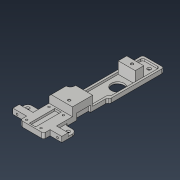
# Autodesk Inventor part: Kameraplatte
Saved by Autodesk Inventor 2022.1 (Build 261234020, 234B)
## iProperties
Part Number: Kameraplatte
Material: Aluminium 6061
Document SubType Name: Modeling
Designer: rYan
Mass: 35.1159 g
Surface Area: 82.272 cm^2
Volume: 13.0059 cm^3
Density: 2.7 g/cm^3
Appearance: Aluminium - flach
Author: rYan
Autodesk Inventor part; units mm, degrees
note: some values were not read from the file. Chosen so that the rebuilt part matches the saved one: direction of "Bohrung4".
ref_plane "YZ Plane" through (0, 0, 0) normal (1, 0, 0) x (0, 1, 0)
ref_plane "XZ Plane" through (0, 0, 0) normal (0, 1, 0) x (-1, 0, 0)
ref_plane "XY Plane" through (0, 0, 0) normal (0, 0, 1) x (1, 0, 0)
sketch "Skizze1" plane through (0, 0, 0) normal (0, 0, 1) x (1, 0, 0)
  line L0 (0, 102.2) -> (0, -102.2) projected
  line L1 (-33.3598, 0) -> (33.3598, 0) projected
  line L2 (14, 73) -> (-10, 73)
  line L3 (14, -73) -> (-10, -73)
  line L4 (-10, -53) -> (-19, -53)
  line L5 (-10, -61) -> (-23, -61)
  arc A0 (-19, -53) -> (-23, -57) centre (-19, -57) ccw
  line L6 (14, -53) -> (19, -53)
  line L7 (14, -61) -> (23, -61)
  arc A1 (23, -57) -> (19, -53) centre (19, -57) ccw
  line L8 (-10, -73) -> (-10, -61)
  line L9 (-10, -53) -> (-10, 73)
  line L10 (14, 73) -> (14, -53)
  line L11 (14, -61) -> (14, -73)
  line L12 (-23, -61) -> (-23, -57)
  line L13 (23, -61) -> (23, -57)
  point P0 (0, 0)
  dimension "d45" = 73
  dimension "d46" = 73
  dimension "d53" = 14
  dimension "d54" = 10
  dimension "d55" = 8
  dimension "d59" = 57
  dimension "d61" = 38
  constraints: 24 end point, 6 tangent, 4 collinear, 4 parallel, 4 point on circle, 3 horizontal, 2 centre point, 2 perpendicular, 2 vertical, 1 symmetric about line
  measures "d45" distance between parallel lines of L2 L1
  measures "d46" distance between parallel lines of L3 L1
  measures "d53" distance between parallel lines of L0 L11
  measures "d54" distance between parallel lines of L8 L0
  measures "d55" distance between parallel lines of L7 L6
  measures "d59" distance from line of L1 A0.centre
  measures "d61" distance of A1.centre A0.centre
extrude "Extrusion1" add sketch "Skizze1" along normal blind 2
sketch "Skizze4" plane through (0, 0, 2) normal (0, 0, 1) x (1, 0, 0)
  line L0 (-10, 73) -> (-10, -53) projected
  line L1 (0, 102.2) -> (0, -102.2) projected
  line L2 (-32.2, 0) -> (32.2, 0) projected
  line L3 (-10, 46) -> (-6, 46)
  line L4 (-6, 46) -> (-6, -30)
  line L5 (-6, -30) -> (-10, -30)
  line L6 (-10, -30) -> (-10, 46)
  line L7 (19, -53) -> (14, -53) projected
  line L8 (14, -53) -> (12, -53)
  line L9 (12, -53) -> (12, -13)
  line L10 (12, -13) -> (14, -13)
  line L11 (14, -13) -> (14, -53)
  line L12 (14, -73) -> (14, -61) projected
  line L13 (-10, -73) -> (14, -73) projected
  line L14 (14, -73) -> (12, -73)
  line L15 (12, -73) -> (12, -61)
  line L16 (12, -61) -> (14, -61)
  line L17 (14, -61) -> (14, -73)
  point P0 (0, 0)
  dimension "d62" = 4
  dimension "d81" = 46
  dimension "d82" = 30
  dimension "d158" = 2
  dimension "d159" = 40
  constraints: 24 end point, 6 parallel, 3 horizontal, 3 perpendicular, 2 point on line, 1 collinear
  measures "d62" distance of L3.start L3.end
  measures "d81" distance between parallel lines of L2 L3
  measures "d82" distance between parallel lines of L5 L2
  measures "d158" distance of L9.end L10.end
  measures "d159" distance of L8.end L9.end
extrude "Extrusion2" cut sketch "Skizze4" against normal through all
sketch "Skizze6" plane through (0, 0, 2) normal (0, 0, 1) x (1, 0, 0)
  line L0 (-6, -30) -> (-10, -30) projected
  line L1 (-10, -30) -> (-10, -53) projected
  line L2 (-10, -53) -> (-19, -53) projected
  arc A0 (-19, -53) -> (-23, -57) centre (-19, -57) ccw projected
  line L3 (-23, -61) -> (-10, -61) projected
  line L4 (-10, -61) -> (-10, -73) projected
  line L5 (-10, -73) -> (12, -73) projected
  line L6 (12, -61) -> (23, -61) projected
  arc A1 (23, -57) -> (19, -53) centre (19, -57) ccw projected
  line L7 (19, -53) -> (12, -53) projected
  line L8 (14, -13) -> (14, 73) projected
  line L9 (14, 73) -> (-10, 73) projected
  line L10 (-10, 73) -> (-10, 46) projected
  line L11 (-10, 46) -> (-6, 46) projected
  line L12 (-6, 46) -> (-6, -30) projected
  line L13 (-10, -73) -> (14, -73) projected
  line L14 (14, -53) -> (14, 73) projected
  line L15 (-10, -73) -> (12, -73)
  line L16 (12, -73) -> (12, -30)
  line L17 (12, -30) -> (-10, -30)
  line L18 (-10, -30) -> (-10, -73)
  line L19 (14, 73) -> (-10, 73) projected
  line L20 (-10, 73) -> (14, 73)
  line L21 (14, 73) -> (14, 46)
  line L22 (14, 46) -> (-10, 46)
  line L23 (-10, 46) -> (-10, 73)
  line L24 (-6, -30) -> (12, -30)
  line L25 (12, -30) -> (12, -27)
  line L26 (12, -27) -> (-6, -27)
  line L27 (-6, -27) -> (-6, -30)
  line L28 (-23, -57) -> (-23, -61) projected
  line L29 (23, -61) -> (23, -57) projected
  line L30 (12, -13) -> (14, -13) projected
  line L31 (12, -53) -> (12, -13) projected
  line L32 (12, -53) -> (12, -13) projected
  line L33 (12, -73) -> (12, -61) projected
  point P0 (0, 0)
  dimension "d83" = 27
  constraints: 24 end point, 6 parallel, 3 horizontal, 3 perpendicular, 3 point on line, 2 collinear
  measures "d83" distance from line of L26 point (0, 0)
extrude "Extrusion3" add sketch "Skizze6" along normal blind 3 contours L17 L16 L5 L4 L18 L1 L0 | L12 L26 L25 L17 | L11 L10 L9 L8 L22
sketch "Skizze7" plane through (0, 0, 5) normal (0, 0, 1) x (1, 0, 0)
  line L0 (12, -27) -> (-6, -27) projected
  line L1 (-6, -27) -> (-6, -30) projected
  line L2 (-6, -30) -> (-10, -30) projected
  line L3 (-10, -30) -> (-10, -73) projected
  line L4 (-10, -73) -> (12, -73) projected
  line L5 (-6, -27) -> (12, -27)
  line L6 (-6, -30) -> (-6, 46) projected
  line L7 (12, -27) -> (-6, -27) projected
  line L8 (12, -27) -> (12, -46)
  line L9 (14, -13) -> (14, 73) projected
  line L10 (12, -46) -> (-10, -46)
  line L11 (-10, -30) -> (-10, -53) projected
  line L12 (-10, -46) -> (-10, -30)
  line L13 (-10, -30) -> (-6, -30) projected
  line L14 (-10, -30) -> (-6, -30)
  line L15 (-6, -30) -> (-6, -27)
  line L16 (12, -73) -> (12, -27) projected
  point P0 (0, 0)
  dimension "d78" = 46
  constraints: 12 end point, 3 perpendicular, 2 collinear, 2 point on line, 1 other
  measures "d78" distance from line of point (0, 0) L10
extrude "Extrusion4" add sketch "Skizze7" along normal blind 8 contours L8 L10 L3 L2 L1 L0
sketch "Skizze8" plane through (0, 0, 2) normal (0, 0, 1) x (1, 0, 0)
  line L0 (14, 46) -> (-6, 46) projected
  line L1 (-6, 46) -> (-6, -27) projected
  line L2 (14, -13) -> (14, 46) projected
  line L3 (-6, -27) -> (12, -27) projected
  line L4 (14, 46) -> (12, 46)
  line L5 (12, 46) -> (12, -13)
  line L6 (12, -13) -> (14, -13)
  line L7 (14, -13) -> (14, 46)
  line L8 (-6, 46) -> (-6, -30) projected
  line L9 (-6, 46) -> (-4, 46)
  line L10 (-4, 46) -> (-4, -27)
  line L11 (-4, -27) -> (-6, -27)
  line L12 (-6, -27) -> (-6, 46)
  line L13 (-10, -53) -> (-19, -53) projected
  arc A0 (-19, -53) -> (-23, -57) centre (-19, -57) ccw projected
  line L14 (-23, -57) -> (-23, -61) projected
  line L15 (-23, -61) -> (-10, -61) projected
  line L16 (12, -61) -> (23, -61) projected
  line L17 (23, -61) -> (23, -57) projected
  arc A1 (23, -57) -> (19, -53) centre (19, -57) ccw projected
  line L18 (19, -53) -> (12, -53) projected
  line L19 (12, -13) -> (14, -13) projected
  line L20 (12, -27) -> (12, -13) projected
  line L21 (-6, -27) -> (12, -27) projected
  line L22 (-10, -61) -> (-10, -53) projected
  line L23 (12, -27) -> (10, -27)
  line L24 (10, -27) -> (10, -11)
  line L25 (10, -11) -> (12, -11)
  line L26 (12, -11) -> (12, -27)
  line L27 (12, -53) -> (12, -61) projected
  point P0 (0, 0)
  dimension "d84" = 2
  dimension "d160" = 2
  dimension "d161" = 2
  dimension "d162" = 2
  constraints: 25 end point, 6 parallel, 3 collinear, 3 horizontal, 3 perpendicular
  measures "d84" distance between parallel lines of L1 L10
  measures "d160" distance between parallel lines of L2 L5
  measures "d161" distance between parallel lines of L25 L6
  measures "d162" distance of L24.end L25.end
extrude "Extrusion5" add sketch "Skizze8" along normal blind 2 contours L2 L6 L5 L0 | L10 L3 L1 L0 | L5 L20 L3 L24 L25
sketch "Skizze2" plane through (0, 0, 2) normal (0, 0, 1) x (1, 0, 0)
  line L0 (-33.3598, 0) -> (33.3598, 0) projected
  line L1 (0, 102.2) -> (0, -102.2) projected
  arc A0 (-19, -53) -> (-23, -57) centre (-19, -57) ccw projected
  arc A1 (23, -57) -> (19, -53) centre (19, -57) ccw projected
  point P0 (0, 0)
  point P1 (6, 32)
  dimension "d50" = 32
  dimension "d60" = 6
  constraints: 2 coincident
  measures "d50" distance from line of point (6, 32) L0
  measures "d60" distance from line of point (6, 32) L1
hole "Bohrung1" at (19, -57, 2) at (6, 32, 2) at (-19, -57, 2) direction (0, 0, -1) diameter 3.3 end through all
sketch "Skizze3" plane through (0, 0, 2) normal (0, 0, 1) x (1, 0, 0)
  line L0 (-7, 70) -> (6.5, 70) construction
  line L1 (6.5, 70) -> (6.5, 49) construction
  line L2 (6.5, 49) -> (-7, 49) construction
  line L3 (-7, 49) -> (-7, 70) construction
  line L4 (-7, -49) -> (6.5, -49) construction
  line L5 (6.5, -49) -> (6.5, -70) construction
  line L6 (6.5, -70) -> (-7, -70) construction
  line L7 (-7, -70) -> (-7, -49) construction
  line L8 (0, 102.2) -> (0, -102.2) projected
  line L9 (-19, -60) -> (19, -60) projected
  line L10 (43, 45) -> (-43, 45) projected
  line L11 (-60.2, 0) -> (60.2, 0) projected
  point P0 (0, 0)
  dimension "d24" = 13.5
  dimension "d25" = 21
  dimension "d26" = 13.5
  dimension "d27" = 21
  dimension "d28" = 7
  dimension "d29" = 7
  dimension "d43" = 49
  constraints: 16 end point, 8 coincident, 4 parallel, 2 horizontal, 2 perpendicular, 1 other
  measures "d24" distance of L1.end L2.end
  measures "d25" distance of L0.end L1.end
  measures "d26" distance of L5.end L6.end
  measures "d27" distance of L4.end L5.end
  measures "d28" distance between parallel lines of L3 L8
  measures "d29" distance between parallel lines of L7 L8
  measures "d43" distance between parallel lines of L11 L4
hole "Bohrung2" at (-7, 70, 2) at (6.5, 70, 2) at (6.5, 49, 2) at (-7, 49, 2) at (-7, -49, 2) at (6.5, -49, 2) at (6.5, -70, 2) at (-7, -70, 2) direction (0, 0, -1) diameter 1.85 end through all both
fillet "Rundung3" radius 2 10 edges at (-10, -73, 2.5) (14, 73, 2.5) (-10, 73, 2.5) (-10, 46, 2.5) (-6, 46, 2) (-6, -30, 6.5) (-10, -30, 6.5) (-10, -53, 1) (12, -73, 2.5) (12, -53, 1)
sketch "Skizze9" plane through (14, -61, 0) normal (0, -1, 0) x (1, 0, 0)
  line L0 (-37, 0) -> (-24, 0) projected
  line L1 (-24, 0) -> (-24, 2) projected
  line L2 (-37, 2) -> (-24, 2) projected
  line L3 (-37, 0) -> (-37, 2) projected
  line L4 (9, 0) -> (9, 2) projected
  line L5 (-24, 5) -> (-22, 5) projected
  line L6 (-37, 0) -> (-24, 0)
  line L7 (-24, 0) -> (-24, 5)
  line L8 (-24, 5) -> (-37, 5)
  line L9 (-37, 5) -> (-37, 0)
  line L10 (9, 0) -> (-2, 0)
  line L11 (-2, 5) -> (9, 5)
  line L12 (9, 5) -> (9, 0)
  line L13 (-2, 0) -> (-2, 5)
  line L14 (9, 0) -> (-2, 0) projected
  line L15 (-2, 2) -> (9, 2) projected
  line L16 (-2, 2) -> (-2, 0) projected
  point P0 (-14, 0)
  dimension "d8" = 0
  constraints: 16 end point, 3 parallel, 2 collinear, 2 horizontal, 1 perpendicular
extrude "Extrusion6" add sketch "Skizze9" along normal blind 6
sketch "Skizze11" plane through (14, -67, 0) normal (0, -1, 0) x (1, 0, 0)
  line L0 (-33, 2) -> (5, 2) construction
  line L1 (-37, 0) -> (-37, 2) projected
  line L2 (-31.35, 0) -> (-34.65, 0) projected
  line L3 (-34.65, 2) -> (-31.35, 2) projected
  line L4 (6.65, 0) -> (3.35, 0) projected
  line L5 (3.35, 2) -> (6.65, 2) projected
  point P0 (-14, 0)
  dimension "d94" = 38
  constraints: 2 end point, 1 horizontal, 1 midpoint, 1 point on line
  measures "d94" distance of L0.start L0.end
hole "Bohrung4" at (19, -67, 2) at (-19, -67, 2) direction (0, 1, 0) diameter 1.85 depth 6
sketch "Skizze12" plane through (0, 0, 2) normal (0, 0, 1) x (1, 0, 0)
  line L0 (0, 102.2) -> (0, -102.2) projected
  line L1 (-32.2, 0) -> (32.2, 0) projected
  point P0 (0, 0)
  point P1 (6, 2.5)
  dimension "d102" = 6
  dimension "d103" = 2.5
  measures "d102" distance from line of point (6, 2.5) L0
  measures "d103" distance from line of point (6, 2.5) L1
hole "Bohrung5" at (6, 2.5, 2) direction (0, 0, -1) diameter 12 end through all
sketch "Skizze13" plane through (0, 0, 5) normal (0, 0, 1) x (1, 0, 0)
  circle A0 centre (-7, 70) radius 0.925 projected
  circle A1 centre (6.5, 70) radius 0.925 projected
  circle A2 centre (6.5, 49) radius 0.925 projected
  circle A3 centre (-7, 49) radius 0.925 projected
  circle A4 centre (6.5, -49) radius 0.925 projected
  circle A5 centre (-7, -49) radius 0.925 projected
  circle A6 centre (-7, -70) radius 0.925 projected
  circle A7 centre (6.5, -70) radius 0.925 projected
  circle A8 centre (6.5, -70) radius 0.925 construction
  line L0 (-7, -49) -> (6.5, -49) construction
  line L1 (6.5, -49) -> (6.5, -70) construction
  line L2 (6.5, -70) -> (-7, -70) construction
  line L3 (-7, -70) -> (-7, -49) construction
  circle A9 centre (-7, 70) radius 0.925 construction
  circle A10 centre (6.5, 49) radius 0.925 construction
  line L4 (-7, 70) -> (6.5, 70) construction
  line L5 (6.5, 70) -> (6.5, 49) construction
  line L6 (6.5, 49) -> (-7, 49) construction
  line L7 (-7, 49) -> (-7, 70) construction
  line L8 (-3, -47.5) -> (3, -47.5)
  line L9 (3, -47.5) -> (3, -71.5)
  line L10 (3, -71.5) -> (-3, -71.5)
  line L11 (-3, -71.5) -> (-3, -47.5)
  line L12 (-3, 71.5) -> (3, 71.5)
  line L13 (3, 71.5) -> (3, 47.5)
  line L14 (3, 47.5) -> (-3, 47.5)
  line L15 (-3, 47.5) -> (-3, 71.5)
  line L16 (0, 102.2) -> (0, -102.2) projected
  point P0 (0, 0)
  dimension "d115" = 1.5
  dimension "d116" = 1.5
  dimension "d117" = 6
  dimension "d118" = 1.5
  dimension "d119" = 1.5
  constraints: 32 end point, 8 parallel, 4 horizontal, 4 perpendicular, 1 point on line, 2 other
  measures "d115" distance between parallel lines of L8 L0
  measures "d116" distance between parallel lines of L10 L2
  measures "d117" distance of L8.start L8.end
  measures "d118" distance between parallel lines of L6 L14
  measures "d119" distance between parallel lines of L12 L4
extrude "Extrusion7" cut sketch "Skizze13" against normal blind 2 contours L8 L16 L10 L11 | L8 L9 L10 L16 | L12 L16 L14 L15 | L12 L13 L14 L16
sketch "Skizze14" plane through (0, 0, 5) normal (0, 0, 1) x (1, 0, 0)
  line L0 (-17.0333, 38) -> (20.6392, 38)
  line L1 (20.6392, 38) -> (20.6392, 88.9456)
  line L2 (20.6392, 88.9456) -> (-17.0333, 88.9456)
  line L3 (-17.0333, 88.9456) -> (-17.0333, 38)
  arc A0 (-6, 44) -> (-8, 46) centre (-8, 44) ccw projected
  point P0 (0, 0)
  dimension "d126" = 6
  constraints: 8 end point, 2 parallel, 1 horizontal, 1 perpendicular
  measures "d126" distance from line of L0 A0.centre
extrude "Extrusion8" cut sketch "Skizze14" against normal through all
sketch "Skizze15" plane through (0, 0, 2) normal (0, 0, 1) x (1, 0, 0)
  line L0 (12, 38) -> (-4, 38) projected
  line L1 (-4, 38) -> (-4, -27) projected
  line L2 (-4, -27) -> (10, -27) projected
  line L3 (12, -11) -> (12, 2.5) projected
  circle A0 centre (6, 2.5) radius 6 projected
  line L4 (12, 2.5) -> (12, 38) projected
  circle A1 centre (6, 32) radius 1.65 projected
  line L5 (12, 2.5) -> (12, 38) projected
  line L6 (-4, 38) -> (-4, -27) projected
  line L7 (12, 38) -> (-4, 38)
  line L8 (-4, 38) -> (-4, 36)
  line L9 (-4, 36) -> (12, 36)
  line L10 (12, 36) -> (12, 38)
  line L11 (12, -51) -> (12, -61) projected
  line L12 (23, -61) -> (23, -57) projected
  arc A2 (23, -57) -> (19, -53) centre (19, -57) ccw projected
  line L13 (19, -53) -> (14, -53) projected
  line L14 (10, -27) -> (10, -11) projected
  line L15 (10, -11) -> (12, -11) projected
  line L16 (12, -61) -> (18.075, -61) projected
  line L17 (18.075, -61) -> (19.925, -61) projected
  line L18 (19.925, -61) -> (23, -61) projected
  arc A3 (12, -51) -> (14, -53) centre (14, -51) ccw projected
  point P0 (0, 0)
  dimension "d123" = 2
  constraints: 8 end point, 2 parallel, 1 horizontal, 1 horizontal alignment, 1 perpendicular, 1 point on line
  measures "d123" distance between parallel lines of L0 L9
extrude "Extrusion9" add sketch "Skizze15" along normal blind 2 contours L4 L9 L1 L0
fillet "Rundung5" radius 2 8 edges at (14, 38, 2) (-6, 38, 2) (-4, 36, 3) (12, 36, 3) (14, -13, 2) (12, -13, 2) (12, -11, 3) (10, -11, 3)
sketch "Skizze18" plane through (12, -53, 2) normal (1, 0, 0) x (0, 0, -1)
  line L0 (2, 21) -> (2, 2) projected
  line L1 (2, 11) -> (-4, 11)
  line L2 (-4, 11) -> (-4, 24)
  line L3 (-4, 24) -> (2, 24)
  line L4 (2, 24) -> (2, 11)
  line L5 (0, 0) -> (2, 0) projected
  line L6 (2, 0) -> (0, 0) projected
  point P0 (2, 53)
  dimension "d164" = 13
  dimension "d165" = 6
  dimension "d192" = 11
  constraints: 8 end point, 2 parallel, 1 horizontal, 1 perpendicular, 1 point on line
  measures "d164" distance of L1.end L2.end
  measures "d165" distance of L2.end L3.end
  measures "d192" distance between parallel lines of L1 L5
extrude "Extrusion10" cut sketch "Skizze18" against normal blind 2
chamfer "Fase3" distance 2 angle 45 1 edges at (10, -35.5, 6)
chamfer "Fase4" distance 0.3 angle 45 4 edges at (19, -55.35, 0) (-19, -55.35, 0) (6, 8.5, 0) (6, 33.65, 0)
sketch "Skizze19" plane through (0, 0, 2) normal (0, 0, 1) x (1, 0, 0)
  arc A0 (11, -10.7321) -> (12, -9) centre (10, -9) ccw projected
  line L0 (12, -9) -> (12, 2.5) projected
  circle A1 centre (6, 2.5) radius 6 projected
  line L1 (12, 2.5) -> (12, 34) projected
  arc A2 (12, 34) -> (10, 36) centre (10, 34) ccw projected
  line L2 (10, 36) -> (-2, 36) projected
  arc A3 (-2, 36) -> (-4, 34) centre (-2, 34) ccw projected
  line L3 (-4, 34) -> (-4, -27) projected
  line L4 (-4, -27) -> (10, -27) projected
  line L5 (10, -27) -> (10, -12.4641) projected
  arc A4 (11, -10.7321) -> (10, -12.4641) centre (12, -12.4641) ccw projected
  circle A5 centre (6, 32) radius 1.65 projected
  line L6 (-4, 34) -> (-4, -27) projected
  line L7 (12, 13) -> (-4, 13)
  line L8 (-4, 13) -> (-4, 21)
  line L9 (-4, 21) -> (12, 21)
  line L10 (12, 21) -> (12, 13)
  point P0 (0, 0)
  dimension "d174" = 8
  dimension "d175" = 13
  constraints: 8 end point, 2 parallel, 2 point on line, 1 horizontal, 1 horizontal alignment, 1 perpendicular
  measures "d174" distance between parallel lines of L9 L7
  measures "d175" distance from line of point (0, 0) L7
extrude "Extrusion11" add sketch "Skizze19" along normal up to surface (11 mm away) contours L7 L3 L9 L1
sketch "Skizze5" plane through (0, 0, 2) normal (0, 0, 1) x (1, 0, 0)
  line L0 (0, 102.2) -> (0, -102.2) projected
  point P0 (0, 0)
  point P1 (0, -33)
  point P2 (0, -40)
  dimension "d66" = 7
  dimension "d67" = 33
  constraints: 2 point on line
  measures "d66" distance of point (0, -40) point (0, -33)
  measures "d67" distance of point (0, 0) point (0, -33)
hole "Bohrung3" [suppressed]
sketch "Skizze20" plane through (0, 0, 13) normal (0, 0, 1) x (1, 0, 0)
  point P0 (0, 0)
  point P1 (5, -42)
  point P2 (5, 17)
  dimension "d178" = 42
  dimension "d179" = 5
  dimension "d180" = 17
  dimension "d181" = 5
  measures "d178" vertical distance of point (5, -42) point (0, 0)
  measures "d179" horizontal distance of point (5, -42) point (0, 0)
  measures "d180" vertical distance of point (5, 17) point (0, 0)
  measures "d181" horizontal distance of point (5, 17) point (0, 0)
hole "Bohrung7" at (5, 17, 13) at (5, -42, 13) direction (0, 0, -1) diameter 1.85 depth 8 countersink diameter 2.5 countersink angle 90
chamfer "Fase5" distance 2 angle 45 4 edges at (-10, -39, 13) (-9.4142, -30.5858, 13) (-8, -30, 13) (-6, -27.5001, 13)
